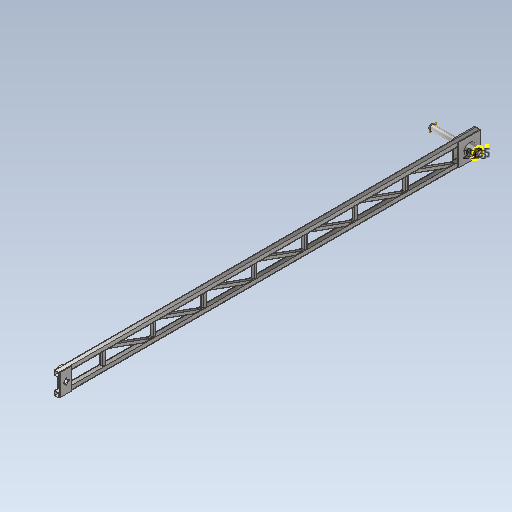
# Autodesk Inventor part: ms truss for link 3
Saved by Autodesk Inventor 2020 (Build 240168000, 168)
## iProperties
Created: 2020-07-27
Part Number: ms truss for link 3
Material: Steel, Mild
Document SubType Name: Modeling
Designer: Vikki
Density: 7.85 g/cm^3
Appearance: Semi-Polished
Mass: 5254.96 g
Surface Area: 7700.9 cm^2
Volume: 669.422 cm^3
Author: Vikki
Autodesk Inventor part; units mm, degrees
ref_plane "YZ Plane" through (0, 0, 0) normal (1, 0, 0) x (0, 1, 0)
ref_plane "XZ Plane" through (0, 0, 0) normal (0, 1, 0) x (-1, 0, 0)
ref_plane "XY Plane" through (0, 0, 0) normal (0, 0, 1) x (1, 0, 0)
sketch "Sketch1" plane through (0, 0, 0) normal (0, 0, 1) x (1, 0, 0)
  line L0 (-9.525, 49.05) -> (9.525, 49.05)
  line L1 (9.525, 49.05) -> (9.525, 30)
  line L2 (9.525, 30) -> (-9.525, 30)
  line L3 (-9.525, 30) -> (-9.525, 49.05)
  line L4 (-9.525, 49.05) -> (9.525, 30) construction
  line L5 (9.525, 49.05) -> (-9.525, 30) construction
  line L6 (-8.325, 47.85) -> (8.325, 47.85)
  line L7 (8.325, 47.85) -> (8.325, 31.2)
  line L8 (8.325, 31.2) -> (-8.325, 31.2)
  line L9 (-8.325, 31.2) -> (-8.325, 47.85)
  line L10 (0, 0) -> (34, 0) construction
  line L11 (-9.525, -49.05) -> (9.525, -49.05)
  line L12 (9.525, -49.05) -> (9.525, -30)
  line L13 (9.525, -30) -> (-9.525, -30)
  line L14 (-9.525, -30) -> (-9.525, -49.05)
  line L15 (-9.525, -49.05) -> (9.525, -30) construction
  line L16 (9.525, -49.05) -> (-9.525, -30) construction
  line L17 (-8.325, -47.85) -> (8.325, -47.85)
  line L18 (8.325, -47.85) -> (8.325, -31.2)
  line L19 (8.325, -31.2) -> (-8.325, -31.2)
  line L20 (-8.325, -31.2) -> (-8.325, -47.85)
  point P0 (0, 39.525)
  point P1 (0, 39.525)
  point P2 (0, -39.525)
  point P3 (0, -39.525)
  dimension "d1" = 19.05
  dimension "d3" = 30
  dimension "d4" = 1.2
  constraints: 42 end point, 10 symmetric about line, 5 midpoint, 4 parallel, 3 perpendicular, 2 horizontal, 1 vertical alignment, 3 other
  measures "d1" distance of L0.start L0.end
  measures "d3" distance from line of L10.start L2
  measures "d4" distance between parallel lines of L2 L8
extrude "Extrusion1" add sketch "Sketch1" along normal blind 1880
sketch "Sketch2" plane through (-9.525, -30, 1880) normal (0, 1, 0) x (1, 0, 0)
  line L0 (19.05, 1880) -> (19.05, 0) projected
  line L1 (19.05, 1880) -> (0, 1880)
  line L2 (0, 1880) -> (0, 1860.95)
  line L3 (0, 1860.95) -> (19.05, 1860.95)
  line L4 (19.05, 1860.95) -> (19.05, 1880)
  line L5 (17.85, 1878.8) -> (1.2, 1878.8)
  line L6 (1.2, 1878.8) -> (1.2, 1862.15)
  line L7 (1.2, 1862.15) -> (17.85, 1862.15)
  line L8 (17.85, 1862.15) -> (17.85, 1878.8)
  point P0 (9.525, 1880)
  point P1 (19.05, 1860.95)
  dimension "d7" = 19.05
  dimension "d8" = 19.05
  dimension "d9" = 1.2
  constraints: 16 end point, 4 parallel, 2 perpendicular, 1 horizontal, 3 other
  measures "d7" distance of L1.end L2.end
  measures "d8" distance of L0.start L1.end
  measures "d9" distance from line of L0.start L8
extrude "Extrusion2" add sketch "Sketch2" along normal up to surface (60 mm away)
sketch "Sketch3" plane through (9.525, -49.05, 0) normal (1, 0, 0) x (0, 0, -1)
  line L0 (0, 0) -> (0, 98.1) projected
  line L1 (0, 98.1) -> (-1880, 98.1) projected
  line L2 (0, 0) -> (-98.1, 0)
  line L3 (-98.1, 0) -> (-98.1, 98.1)
  line L4 (-98.1, 98.1) -> (0, 98.1)
  line L5 (0, 98.1) -> (0, 0)
  circle A0 centre (-49.05, 49.05) radius 15
  point P0 (0, 49.05)
  dimension "d17" = 49.05
  dimension "d18" = 49.05
  dimension "d68" = 30
  constraints: 8 end point, 2 parallel, 2 perpendicular, 1 centre point, 1 horizontal, 1 point on line
  measures "d17" distance from line of L1 A0.centre
  measures "d18" distance from line of L0 A0.centre
  measures "d68" diameter of A0
extrude "Extrusion3" add sketch "Sketch3" along normal blind 4
sketch "Sketch4" plane through (-9.525, -49.05, 0) normal (-1, 0, 0) x (0, 0, 1)
  line L0 (0, 98.1) -> (98.1, 98.1) projected
  line L1 (98.1, 98.1) -> (98.1, 0) projected
  line L2 (98.1, 0) -> (0, 0) projected
  line L3 (0, 0) -> (0, 98.1) projected
  circle A0 centre (49.05, 49.05) radius 15 projected
  point P0 (0, 49.05)
extrude "Extrusion4" add sketch "Sketch4" along normal blind 4
sketch "Sketch5" plane through (13.525, -49.05, 0) normal (1, 0, 0) x (0, 0, -1)
  circle A0 centre (-49.05, 49.05) radius 15 projected
  circle A1 centre (-49.05, 49.05) radius 25
  point P0 (0, 49.05)
  dimension "d19" = 50
  constraints: 1 centre point, 1 coincident
  measures "d19" diameter of A1
extrude "Extrusion5" add sketch "Sketch5" along normal blind 30
sketch "Sketch6" plane through (9.525, -30, 1880) normal (0, 1, 0) x (1, 0, 0)
  line L0 (-15.875, 1733.3338) -> (-3.175, 1733.3338)
  line L1 (-3.175, 1733.3338) -> (-3.175, 1770.4661)
  line L2 (-3.175, 1770.4661) -> (-15.875, 1770.4661)
  line L3 (-15.875, 1770.4661) -> (-15.875, 1733.3338)
  line L4 (-15.875, 1733.3338) -> (-3.175, 1770.4661) construction
  line L5 (-3.175, 1733.3338) -> (-15.875, 1770.4661) construction
  line L6 (0, 1781.9) -> (0, 0) projected
  line L7 (-3.975, 1769.6662) -> (-3.975, 1734.1339)
  line L8 (-3.975, 1734.1339) -> (-15.075, 1734.1339)
  line L9 (-15.075, 1734.1339) -> (-15.075, 1769.6662)
  line L10 (-15.075, 1769.6662) -> (-3.975, 1769.6662)
  point P0 (-9.525, 1880)
  point P1 (-9.525, 1751.9)
  dimension "d22" = 9.525
  dimension "d23" = 30
  dimension "d24" = 12.7
  dimension "d26" = 37.1323
  dimension "d27" = 0.8
  constraints: 20 end point, 5 parallel, 2 midpoint, 1 horizontal, 3 other
  measures "d22" distance from line of point (-9.525, 1751.9) L6
  measures "d23" vertical distance of point (-9.525, 1751.9) L6.start
  measures "d24" distance of L1.end L2.end
  measures "d26" distance of L0.end L1.end
  measures "d27" distance between parallel lines of L1 L7
sketch "Sketch7" plane through (9.525, 30, 98.1) normal (0, -1, 0) x (1, 0, 0)
  line L0 (-9.525, 30) -> (-9.525, 194.8486) construction
  point P0 (-9.525, -98.1)
  dimension "d28" = 164.8486
  constraints: 2 end point, 1 vertical
  measures "d28" distance of L0.start L0.end
sketch3d "3D Sketch1"
  line L0 (0, -30, 128.1) -> (0, 30, 292.9486)
sweep "Sweep1" add profiles "Sketch6" path "3D Sketch1"
sketch "Sketch8" plane through (9.525, 30, 98.1) normal (0, -1, 0) x (1, 0, 0)
  line L0 (-3.175, 231.1148) -> (-15.875, 231.1148)
  line L1 (-15.875, 231.1148) -> (-15.875, 218.4148)
  line L2 (-15.875, 218.4148) -> (-3.175, 218.4148)
  line L3 (-3.175, 218.4148) -> (-3.175, 231.1148)
  line L4 (-15.875, 176.2824) -> (-15.875, 213.4148) projected
  line L5 (-3.175, 213.4148) -> (-3.175, 176.2824) projected
  line L6 (-15.875, 213.4148) -> (-3.175, 213.4148) projected
  line L7 (-15.075, 230.3148) -> (-3.975, 230.3148)
  line L8 (-3.975, 230.3148) -> (-3.975, 219.2148)
  line L9 (-3.975, 219.2148) -> (-15.075, 219.2148)
  line L10 (-15.075, 219.2148) -> (-15.075, 230.3148)
  point P0 (-9.525, -98.1)
  dimension "d31" = 5
  dimension "d32" = 0.8
  constraints: 16 end point, 4 parallel, 3 perpendicular, 2 collinear, 1 horizontal, 3 other
  measures "d31" distance between parallel lines of L2 L6
  measures "d32" distance between parallel lines of L1 L10
extrude "Extrusion6" add sketch "Sketch8" along normal up to surface (60 mm away)
sketch "Sketch9" plane through (13.525, -49.05, 0) normal (1, 0, 0) x (0, 0, -1)
  circle A0 centre (-1849.05, 49.05) radius 7.5
  circle A1 centre (-49.05, 49.05) radius 15 projected
  line L0 (0, 1.2) -> (-1880, 1.2) projected
  line L1 (-98.1, 98.1) -> (-1880, 98.1) projected
  line L2 (-1874.05, 1.2) -> (-1824.05, 1.2)
  line L3 (-1824.05, 1.2) -> (-1824.05, 98.1)
  line L4 (-1824.05, 98.1) -> (-1874.05, 98.1)
  line L5 (-1874.05, 98.1) -> (-1874.05, 1.2)
  point P0 (0, 49.05)
  dimension "d35" = 15
  dimension "d36" = 1800
  dimension "d40" = 50
  dimension "d41" = 25
  constraints: 8 end point, 2 parallel, 2 point on line, 1 centre point, 1 horizontal, 1 horizontal alignment, 1 perpendicular
  measures "d35" diameter of A0
  measures "d36" distance of A0.centre A1.centre
  measures "d40" distance of L3.end L4.end
  measures "d41" distance from line of L5 A0.centre
pattern_linear "Rectangular Pattern1" count 7 spacing 225 along (0, 0, 1) of "Sweep1", "Extrusion6"
extrude "Extrusion7" add sketch "Sketch9" against normal blind 4 contours L0 L5 L1 L3
sketch "Sketch11" plane through (-9.525, 30, 98.1) normal (-1, 0, 0) x (0, 0, 1)
  line L0 (1725.95, -77.85) -> (1725.95, 19.05) projected
  line L1 (1725.95, 19.05) -> (1775.95, 19.05) projected
  line L2 (1775.95, 19.05) -> (1775.95, -77.85) projected
  line L3 (1775.95, -77.85) -> (1725.95, -77.85) projected
  circle A0 centre (1750.95, -30) radius 7.5 projected
  line L4 (1738.45, -77.85) -> (1738.45, 19.05)
  line L5 (1763.45, -77.85) -> (1763.45, 19.05)
  line L6 (0, 19.05) -> (1781.9, 19.05) projected
  point P0 (-98.1, -30)
  point P1 (1763.45, 19.05)
  dimension "d75" = 12.5
  dimension "d76" = 12.5
  constraints: 4 end point, 4 point on line, 2 parallel, 1 perpendicular
  measures "d75" distance from line of A0.centre L4
  measures "d76" distance from line of A0.centre L5
extrude "Extrusion9" add sketch "Sketch11" along normal blind 4 contours L4 L1 L5 L3
sketch "Sketch12" plane through (-13.525, -49.05, 0) normal (-1, 0, 0) x (0, 0, 1)
  circle A0 centre (49.05, 49.05) radius 15 projected
  circle A1 centre (49.05, 49.05) radius 25
  point P0 (0, 49.05)
  dimension "d48" = 50
  constraints: 1 centre point, 1 coincident
  measures "d48" diameter of A1
extrude "Extrusion10" cut sketch "Sketch12" against normal blind 1
sketch "Sketch13" plane through (9.525, -30, 98.1) normal (0, 1, 0) x (1, 0, 0)
  line L0 (0, 0) -> (0, -1781.9) projected
  line L1 (0, -1762.85) -> (-19.05, -1762.85)
  line L2 (-19.05, -1762.85) -> (-19.05, -1781.9)
  line L3 (-19.05, -1781.9) -> (0, -1781.9)
  line L4 (0, -1781.9) -> (0, -1762.85)
  line L5 (-1.2, -1780.7) -> (-17.85, -1780.7)
  line L6 (-17.85, -1780.7) -> (-17.85, -1764.05)
  line L7 (-17.85, -1764.05) -> (-1.2, -1764.05)
  line L8 (-1.2, -1764.05) -> (-1.2, -1780.7)
  point P0 (-9.525, 98.1)
  dimension "d51" = 19.05
  dimension "d52" = 19.05
  dimension "d53" = 1.2
  constraints: 16 end point, 4 parallel, 2 perpendicular, 1 horizontal, 1 point on line, 3 other
  measures "d51" distance between parallel lines of L3 L1
  measures "d52" distance of L2.end L0.end
  measures "d53" distance between parallel lines of L3 L5
extrude "Extrusion11" [suppressed]
sketch "Sketch14" plane through (-13.525, 30, 98.1) normal (-1, 0, 0) x (0, 0, 1)
  circle A0 centre (1750.95, -30) radius 7.5 projected
  circle A1 centre (1750.95, -30) radius 7.5 projected
  circle A2 centre (1750.95, -30) radius 12.5
  point P0 (-98.1, -30)
  dimension "d56" = 25
  constraints: 1 centre point, 1 coincident
  measures "d56" diameter of A2
extrude "Extrusion12" cut sketch "Sketch14" against normal blind 1
sketch "Sketch15" plane through (13.525, -49.05, 0) normal (1, 0, 0) x (0, 0, -1)
  circle A0 centre (-1849.05, 49.05) radius 7.5 projected
  line L0 (-1849.05, 49.05) -> (-1849.05, 36.05)
  circle A1 centre (-1849.05, 36.05) radius 1.5
  line L1 (-1824.05, 1.2) -> (-1824.05, 98.1) projected
  circle A2 centre (-1836.05, 49.05) radius 1.5
  circle A3 centre (-1849.05, 62.05) radius 1.5
  circle A4 centre (-1862.05, 49.05) radius 1.5
  circle A5 centre (-1849.05, 49.05) radius 7.5 projected
  circle A6 centre (-1849.05, 49.05) radius 10
  point P0 (0, 49.05)
  dimension "d59" = 13
  dimension "d60" = 3
  dimension "d63" = 360
  dimension "d65" = 20
  constraints: 5 centre point, 2 coincident, 2 end point, 1 parallel, 1 vertical, 9 other
  measures "d59" distance of L0.start L0.end
  measures "d60" diameter of A1
  measures "d65" diameter of A6
extrude "Extrusion13" cut sketch "Sketch15" against normal blind 4
sketch "Sketch17" plane through (-12.525, 0, 49.05) normal (-1, 0, 0) x (0, 0, 1)
  circle A0 centre (0, 0) radius 25 projected
  circle A1 centre (0, 0) radius 15 projected
  point P0 (-49.05, 0)
extrude "Extrusion15" add sketch "Sketch17" along normal blind 14
sketch "Sketch19" plane through (43.525, 0, 49.05) normal (1, 0, 0) x (0, 0, -1)
  circle A0 centre (0, 0) radius 15 projected
  circle A1 centre (0, 0) radius 25 projected
  circle A2 centre (0, 0) radius 25 projected
  circle A3 centre (0, 0) radius 14.75
  line L0 (14.4914, -2.75) -> (19.75, -2.75)
  line L1 (19.75, -2.75) -> (19.75, 2.75)
  line L2 (19.75, 2.75) -> (14.4914, 2.75)
  arc A4 (14.4914, 2.75) -> (14.4914, -2.75) centre (0, 0) ccw
  line L3 (19.75, -2.75) -> (19.75, 2.75)
  line L4 (19.75, 2.75) -> (7.25, 2.75)
  line L5 (7.25, 2.75) -> (7.25, -2.75)
  line L6 (7.25, -2.75) -> (19.75, -2.75)
  line L7 (20, 3) -> (20, -3) projected
  line L8 (20, -3) -> (20, 3)
  line L9 (20, 3) -> (7, 3)
  line L10 (7, 3) -> (7, -3)
  line L11 (7, -3) -> (20, -3)
  point P0 (49.05, 0)
  point P1 (14.4417, 3)
  point P2 (14.4417, -3)
  point P3 (14.4914, -2.75)
  point P4 (14.4914, 2.75)
  dimension "d77" = 29.5
  dimension "d79" = 0.25
  dimension "d80" = 12.5
  constraints: 22 end point, 5 equal length, 2 centre point, 2 perpendicular, 2 point on circle, 1 coincident
  measures "d77" diameter of A3
  measures "d79" distance between parallel lines of L10 L5
  measures "d80" distance between parallel lines of L5 L1
sketch "Sketch24" plane through (43.525, 0, 49.05) normal (1, 0, 0) x (0, 0, -1)
  circle A0 centre (0, 0) radius 15 projected
  circle A1 centre (0, 0) radius 12.75
  point P0 (49.05, 0)
  dimension "d97" = 25.5
  constraints: 1 centre point, 1 coincident
  measures "d97" diameter of A1
extrude "Extrusion20" add sketch "Sketch24" against normal up to surface (57.05 mm away)
sketch "Sketch25" plane through (43.525, 0, 49.05) normal (1, 0, 0) x (0, 0, -1)
  circle A0 centre (0, 0) radius 12.75 projected
  circle A1 centre (0, 0) radius 12.5
  point P0 (49.05, 0)
  dimension "d100" = 25
  constraints: 1 centre point, 1 coincident
  measures "d100" diameter of A1
extrude "Extrusion21" add sketch "Sketch25" along normal blind 15 and the other way blind 200 contours A1
sketch "Sketch26" plane through (43.525, 0, 49.05) normal (1, 0, 0) x (0, 0, -1)
  point P0 (49.05, 0)
sketch "Sketch27" plane through (43.525, 0, 49.05) normal (1, 0, 0) x (0, 0, -1)
  line L0 (4, -15.8) -> (-4, -15.8)
  circle A0 centre (0, 0) radius 12.5 projected
  line L1 (-4, -15.8) -> (-4, -11.8427)
  circle A1 centre (0, 0) radius 12.5 projected
  line L2 (4, -15.8) -> (4, -11.8427)
  point P0 (49.05, 0)
  point P1 (-4, -11.8427)
  dimension "d105" = 8
  dimension "d106" = 15.8
  dimension "d107" = 4
  constraints: 6 end point, 1 horizontal, 1 parallel, 1 vertical, 4 other
  measures "d105" distance of L0.start L0.end
  measures "d106" distance from line of point (0, 0) L0
  measures "d107" horizontal distance of L0.start point (0, 0)
extrude "Extrusion22" cut sketch "Sketch27" against normal blind 20 contours L0 L1 A0 L2
ref_plane "Work Plane3" through (50.775, 0, 49.05) normal (1, 0, 0) x (0, 0, -1)
sketch "Sketch28" plane through (50.775, 0, 49.05) normal (1, 0, 0) x (0, 0, -1)
  circle A0 centre (0, 0) radius 12.5 projected
  circle A1 centre (0, 0) radius 14
  point P0 (49.05, 0)
  dimension "d111" = 28
  constraints: 1 centre point, 1 coincident
  measures "d111" diameter of A1
extrude "Extrusion23" add sketch "Sketch28" along normal blind 2
ref_plane "Work Plane4" through (-150.475, 0, 49.05) normal (-1, 0, 0) x (0, 0, 1)
sketch "Sketch29" plane through (-150.475, 0, 49.05) normal (-1, 0, 0) x (0, 0, 1)
  circle A0 centre (0, 0) radius 12.5 projected
  circle A1 centre (0, 0) radius 14
  point P0 (-49.05, 0)
  dimension "d115" = 28
  constraints: 1 centre point, 1 coincident
  measures "d115" diameter of A1
extrude "Extrusion24" add sketch "Sketch29" along normal blind 2
equation "\"d7\" = d1"
equation "\"d8\" = d1"
equation "\"d22\" = 0.5 * d1"
equation "\"d52\" = d1"
body "Solid1"
